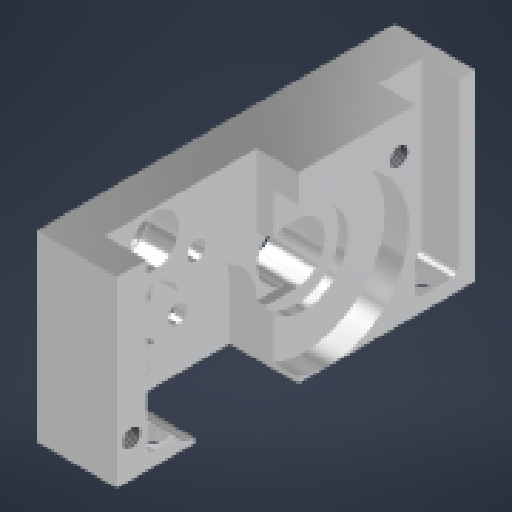
# Autodesk Inventor part: MocowanieLewejPrzekladni
Saved by Autodesk Inventor 2023 (Build 270158000, 158)
## iProperties
Created: 2022-03-16
Part Number: MocowanieLewejPrzekladni
Material: Aluminium 6061
Document SubType Name: Modeling
Designer: Michał
Density: 2.7 g/cm^3
Appearance: Aluminium — płaski
Mass: 20.1298 g
Surface Area: 53.9429 cm^2
Volume: 7.45546 cm^3
Author: Michał
Autodesk Inventor part; units mm, degrees
ref_plane "YZ Plane" through (0, 0, 0) normal (1, 0, 0) x (0, 1, 0)
ref_plane "XZ Plane" through (0, 0, 0) normal (0, 1, 0) x (-1, 0, 0)
ref_plane "XY Plane" through (0, 0, 0) normal (0, 0, 1) x (1, 0, 0)
sketch "Szkic1" plane through (0, 0, 0) normal (1, 0, 0) x (0, 1, 0)
  line L0 (0, 0) -> (25, 0)
  line L1 (25, 0) -> (25, -49)
  line L2 (25, -49) -> (0, -49)
  line L3 (0, -49) -> (0, 0)
  dimension "dlugosc" = 49
  dimension "wysokosc" = 25
  constraints: 8 end point, 2 parallel, 1 horizontal, 1 perpendicular
  measures "dlugosc" distance of L0.end L1.end
  measures "wysokosc" distance of L1.end L2.end
extrude "Wyciągnięcie proste1" add sketch "Szkic1" along normal blind 11
sketch "Szkic2" plane through (11, 0, 0) normal (1, 0, 0) x (0, 0, -1)
  circle A0 centre (10.8, 12.5) radius 3.5
  circle A1 centre (16.5416, 17.0276) radius 1.25
  circle A2 centre (17.6791, 7.0925) radius 1.25
  line L0 (0, 25) -> (0, 0) construction
  line L1 (16.5416, 17.0276) -> (28.9, 11) construction
  line L2 (28.9, 11) -> (28.9, 0) construction
  line L3 (49, 25) -> (0, 25) construction
  line L4 (49, 0) -> (49, 25) projected
  line L5 (40.8, 25) -> (46.7, 25)
  line L6 (46.7, 25) -> (46.7, 2)
  line L7 (40.8, 25) -> (40.8, 2)
  line L8 (40.8, 2) -> (46.7, 2)
  line L9 (0, 0) -> (49, 0) projected
  line L10 (4.05, 25) -> (9.95, 25)
  line L11 (9.95, 25) -> (9.95, 2)
  line L12 (9.95, 2) -> (4.05, 2)
  line L13 (4.05, 2) -> (4.05, 25)
  point P0 (2, 5)
  point P1 (38.5, 20)
  point P2 (7, 25)
  point P3 (43.75, 25)
  dimension "d4" = 2.5
  dimension "d5" = 7
  dimension "Odl01" = 8.75
  dimension "Odl12" = 10
  dimension "d8" = 10.8
  dimension "d10" = 13.75
  dimension "d11" = 28.9
  dimension "d13" = 64
  dimension "d53" = 2
  dimension "d85" = 2
  dimension "d86" = 5.9
  dimension "d87" = 12.5
  dimension "d88" = 11
  dimension "d89" = 7
  dimension "d107" = 5.25
  dimension "d108" = 5
  dimension "d109" = 10.5
  dimension "d113" = 5
  constraints: 20 end point, 3 centre point, 3 horizontal, 3 point on line, 2 collinear, 2 midpoint, 2 parallel, 2 perpendicular, 2 vertical, 1 equal radius
  measures "d4" diameter of A1
  measures "d5" diameter of A0
  measures "Odl01" distance of A2.centre A0.centre
  measures "Odl12" distance of L1.start A2.centre
  measures "d8" distance from line of L0 A0.centre
  measures "d10" distance of L1.end L1.start
  measures "d11" distance from line of L0 L1.end
  measures "d13" angle of L2 L1
  measures "d53" distance from line of L0 point (2, 5)
  measures "d85" distance between parallel lines of L9 L8
  measures "d86" distance between parallel lines of L6 L7
  measures "d87" distance from line of L9 A0.centre
  measures "d88" distance of L1.end L2.end
  measures "d89" distance from line of L0 point (7, 25)
  measures "d107" distance from line of L4 point (43.75, 25)
  measures "d108" distance from line of L3 point (38.5, 20)
  measures "d109" distance from line of L4 point (38.5, 20)
  measures "d113" distance from line of L9 point (2, 5)
extrude "Wyciągnięcie proste2" cut sketch "Szkic2" against normal through all contours A0 L11 | L11 A0 | A1 | A2
hole "Otwór1" at (11, 11, -28.9) direction (-1, 0, 0) diameter 8.1 end through all
hole "Otwór2" at (11, 7.0925, -17.6791) direction (-1, 0, 0) diameter 14 depth 9.4
hole "Otwór3" at (11, 17.0276, -16.5416) direction (-1, 0, 0) diameter 16.5 depth 5.8
sketch "Szkic3" plane through (11, 0, 0) normal (1, 0, 0) x (0, 0, -1)
  circle A0 centre (10.8, 12.5) radius 3.5 construction
  line L0 (10.8, 12.5) -> (10.8, 4) construction
  line L1 (10.8, 12.5) -> (10.8, 21) construction
  point P0 (0, 0)
  dimension "d37" = 8.5
  constraints: 4 end point, 2 vertical, 1 collinear
  measures "d37" distance of L0.start L0.end
hole "Otwór4" at (11, 4, -10.8) at (11, 21, -10.8) direction (-1, 0, 0) diameter 6.8 depth 9.5
sketch "Szkic4" plane through (1.5, 21, -10.8) normal (1, 0, 0) x (0, 0, -1)
  arc A0 (-0.1143, -13.6019) -> (2.4657, -19.341) centre (0, -17) ccw projected
  arc A1 (-2.3653, -2.4424) -> (1.4517, 3.0745) centre (0, 0) ccw projected
  point P0 (-10.8, -21)
  point P1 (0, -17)
  constraints: 2 coincident
hole "Otwór5" at (1.5, 21, -10.8) at (1.5, 4, -10.8) direction (-1, 0, 0) diameter 3.4 depth 5.2 countersink diameter 6.3 countersink angle 90 clearance for "Śruba ze łbem stożkowym ISO 2009/7046" size "M3" standard "ISO"
hole "Otwór6" at (11, 5, -2) at (11, 20, -38.5) direction (-1, 0, 0) diameter 2.459 end through all thread size "M3x0.5" class "6H" standard "ISO Metric profile"
hole "Otwór7" at (11, 11, -28.9) direction (-1, 0, 0) diameter 22 depth 3.3
extrude "Wyciągnięcie proste3" cut sketch "Szkic2" against normal blind 5 contours L11 A0 | A0 L11 L12 L13 L10 | L5 L6 L8 L7 picked at (8.7482, 13.1611)
sketch "Szkic6" plane through (0, 0, -49) normal (0, 0, -1) x (-1, 0, 0)
  line L0 (0, 25) -> (0, 0) projected
  line L1 (0, 0) -> (-11, 0) projected
  point P0 (-4, 5)
  point P1 (-4, 17)
  dimension "d90" = 4
  dimension "d91" = 5
  dimension "d92" = 17
  constraints: 1 vertical alignment
  measures "d90" distance from line of point (-4, 17) L0
  measures "d91" distance from line of point (-4, 5) L1
  measures "d92" distance from line of L1 point (-4, 17)
hole "Otwór9" at (4, 17, -49) at (4, 5, -49) direction (0, 0, 1) diameter 2.459 depth 7 tip angle 118 thread size "M3x0.5" class "6H" standard "ISO Metric profile"
sketch "Szkic7" plane through (11, 2, -40.8) normal (0, 1, 0) x (1, 0, 0)
  line L0 (-2.05, 2.95) -> (-5, 2.95) construction
  line L1 (-5, 0) -> (-5, 5.9) construction
  line L2 (-2.05, 2.95) -> (-2.05, 5.9) construction
  line L3 (-2.05, 2.95) -> (-2.05, 0) construction
  line L4 (0, 0) -> (-5, 0) construction
  line L5 (-2.05, -33.8) -> (-2.05, -36.75) construction
  line L6 (0, -36.75) -> (-5, -36.75) construction
  line L7 (-2.05, -33.8) -> (-5, -33.8) construction
  line L8 (-5, -32.7495) -> (-5, -36.75) construction
  line L9 (-2.05, -33.8) -> (-2.05, -30.85) construction
  line L10 (0, -30.85) -> (-5, -30.85) construction
  line L11 (0, 5.9) -> (-5, 5.9) projected
  point P0 (-11, -40.8)
  constraints: 12 end point, 6 point on line, 5 perpendicular, 3 vertical, 1 horizontal, 1 midpoint
hole "Otwór10" at (8.95, 2, -7) at (8.95, 2, -43.75) direction (0, -1, 0) diameter 3.2 end through all clearance for "Śruba ze łbem stożkowym ISO 2009/7046" size "M3" standard "ISO"
fillet "Zaokrąglenie1" radius 1 3 edges at (8.5, 2, -40.8) (8.5, 2, -46.7) (8.5, 2, -4.05)
sketch "Szkic8" plane through (11, 0, 0) normal (1, 0, 0) x (0, 0, -1)
  line L0 (9.95, 9.1048) -> (9.95, 7.292) projected
  arc A0 (9.95, 9.1048) -> (10.9448, 9.003) centre (10.8, 12.5) ccw projected
  arc A1 (10.9448, 9.003) -> (10.6857, 7.3981) centre (17.6791, 7.0925) ccw projected
  arc A2 (10.6857, 7.3981) -> (9.95, 7.292) centre (10.8, 4) ccw projected
  arc A3 (12.2517, 24.0745) -> (9.95, 24.292) centre (10.8, 21) ccw projected
  arc A4 (14.4195, 25) -> (12.2517, 24.0745) centre (16.5416, 17.0276) ccw projected
  line L1 (14.4195, 25) -> (9.95, 25) projected
  line L2 (9.95, 25) -> (9.95, 24.292) projected
  arc A5 (4.05, 3) -> (5.05, 2) centre (5.05, 3) ccw projected
  line L3 (8.0505, 2) -> (5.05, 2) projected
  arc A6 (9.95, 7.292) -> (8.0505, 2) centre (10.8, 4) ccw projected
  line L4 (9.95, 9.1048) -> (9.95, 7.292) projected
  arc A7 (8.509, 15.146) -> (9.95, 9.1048) centre (10.8, 12.5) ccw projected
  arc A8 (8.4347, 18.5576) -> (8.509, 15.146) centre (16.5416, 17.0276) ccw projected
  arc A9 (9.95, 24.292) -> (8.4347, 18.5576) centre (10.8, 21) ccw projected
  line L5 (9.95, 25) -> (9.95, 24.292) projected
  line L6 (4.05, 25) -> (9.95, 25) projected
  line L7 (4.05, 3) -> (4.05, 25) projected
  arc A10 (22.8933, 11.7628) -> (23.8839, 20.7897) centre (16.5416, 17.0276) ccw projected
  arc A11 (23.8839, 20.7897) -> (18.6637, 25) centre (16.5416, 17.0276) ccw projected
  line L8 (16.5416, 17.0276) -> (24.7916, 17.0276) construction
  line L9 (24.7916, 17.0276) -> (24.7916, 25)
  line L10 (24.7916, 25) -> (18.6637, 25)
  line L11 (24.7916, 17.0276) -> (24.7916, 0)
  line L12 (0, 0) -> (28.9, 0) projected
  arc A12 (8.0505, 2) -> (13.2657, 1.659) centre (10.8, 4) ccw projected
  line L13 (13.2657, 1.659) -> (13.2657, 0)
  line L14 (8.0505, 2) -> (5.05, 2) projected
  line L15 (8.0505, 2) -> (13.2657, 2)
  line L16 (13.2657, 2) -> (13.2657, 1.659)
  arc A13 (22.8933, 11.7628) -> (14.2323, 13.1851) centre (17.6791, 7.0925) ccw projected
  line L17 (13.2657, 2) -> (22.8933, 11.7628)
  line L18 (24.7916, 0) -> (13.2657, 0)
  constraints: 18 end point, 3 perpendicular, 2 horizontal, 2 point on line, 1 collinear, 1 point on circle, 1 tangent, 1 vertical
extrude "Wyciągnięcie proste4" cut sketch "Szkic8" against normal up to surface (5.8 mm away) contours A0 A1 A2 L0 | A10 A11 L10 L9 | L0 A6 L3 A5 L7 L6 L2 A9 A8 A7 | L16 L17 A10 L11 L12 L13 | L2 L1 A4 A3
sketch "Szkic13" plane through (11, 0, 0) normal (1, 0, 0) x (0, 0, -1)
  circle A0 centre (17.6791, 7.0925) radius 1.25 projected
  arc A1 (13.2657, 1.659) -> (10.6857, 7.3981) centre (10.8, 4) ccw projected
  arc A2 (13.2657, 1.659) -> (14.2323, 13.1851) centre (17.6791, 7.0925) ccw projected
  arc A3 (10.9448, 9.003) -> (14.2323, 13.1851) centre (10.8, 12.5) ccw projected
  arc A4 (10.9448, 9.003) -> (10.6857, 7.3981) centre (17.6791, 7.0925) ccw projected
  arc A5 (13.2657, 1.659) -> (14.2323, 13.1851) centre (17.6791, 7.0925) ccw projected
  line L0 (24.7916, 0) -> (24.7916, 25) projected
  line L1 (24.7916, 0) -> (13.2657, 0) projected
  line L2 (24.7916, 0) -> (10.6791, 0)
  line L3 (10.6791, 0) -> (10.6791, 7.0925)
  arc A6 (10.9448, 9.003) -> (10.6857, 7.3981) centre (17.6791, 7.0925) ccw projected
  circle A7 centre (17.6791, 7.0925) radius 7
  line L4 (17.6791, 14.0925) -> (24.7916, 14.0925)
  point P0 (0, 0)
  constraints: 6 end point, 3 point on circle, 2 tangent, 1 centre point, 1 coincident, 1 collinear, 1 perpendicular, 1 point on line, 1 vertical
extrude "Wyciągnięcie proste7" cut sketch "Szkic13" against normal up to surface (9.4 mm away)
fillet "Zaokrąglenie2" radius 7 1 edges at (3.4, 14.0925, -24.7916)
sketch "Sketch14" plane through (7.7, 0.796, -24.7916) normal (1, 0, 0) x (0, 0, -1)
  circle A0 centre (4.1084, 10.204) radius 4.05 projected
  circle A1 centre (4.1084, 10.204) radius 6
  point P0 (-24.7916, -0.796)
  dimension "d123" = 12
  constraints: 1 centre point, 1 coincident
  measures "d123" diameter of A1
extrude "Extrusion8" cut sketch "Sketch14" against normal blind 1.2
sketch "Sketch15" plane through (6.5, 0.796, -24.7916) normal (1, 0, 0) x (0, 0, -1)
  circle A0 centre (4.1084, 10.204) radius 4.05 projected
  line L0 (4.1084, 6.154) -> (0, 6.154)
  line L1 (0, 6.154) -> (0, 14.254)
  line L2 (0, 14.254) -> (4.1084, 14.254)
  line L3 (0, 5.8312) -> (0, 14.5767) construction
  point P0 (-24.7916, -0.796)
  constraints: 6 end point, 2 horizontal, 2 point on circle, 2 tangent, 1 collinear
extrude "Extrusion9" cut sketch "Sketch15" along normal up to surface (1.3 mm away) from surface at -1.3 contours A0 L0 L1 L2
